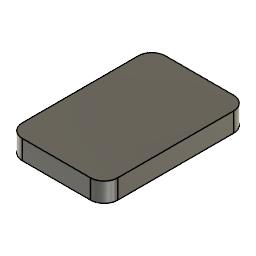
NarBot_asm (Autodesk Fusion 360 archive; units mm, degrees)
design "akupank"
part number: 2026-06-09-16-47-08-805
Autodesk Fusion 360 part; units mm, degrees
sketch "Sketch1" plane through (0, 0, 0) normal (0, 0, 1) x (1, 0, 0)
  line L0 (0, 0) -> (70, 0)
  line L1 (70, 0) -> (70, 105)
  line L2 (70, 105) -> (0, 105)
  line L3 (0, 105) -> (0, 0)
  dimension "d1" = 105
  dimension "d2" = 70
  constraint horizontal L0
  constraint vertical L1
  constraint horizontal L2
  constraint vertical L3
  constraint coincident L0.start L3.end
  measures "d1" distance of L0.start L2.end
  measures "d2" distance of L0.start L0.end
extrude "Extrude1" add sketch "Sketch1" along normal blind 14.2
fillet "Fillet1" radius 10 4 edges at (70, 0, 7.1) (0, 0, 7.1) (70, 105, 7.1) (0, 105, 7.1)
